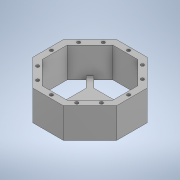
# Autodesk Inventor part: Base_Mount
Saved by Autodesk Inventor 2022 (Build 260153000, 153)
## iProperties
Created: 2022-03-21
Part Number: Base_Mount
Material: Generic
Document SubType Name: Modeling
Designer: Mlees
Density: 1 g/cm^3
Appearance: Smooth - Medium Gray
Author: Mlees
Autodesk Inventor part; units mm, degrees
ref_plane "YZ Plane" through (0, 0, 0) normal (1, 0, 0) x (0, 1, 0)
ref_plane "XZ Plane" through (0, 0, 0) normal (0, 1, 0) x (-1, 0, 0)
ref_plane "XY Plane" through (0, 0, 0) normal (0, 0, 1) x (1, 0, 0)
sketch "Sketch1" plane through (0, 0, 0) normal (0, 1, 0) x (-1, 0, 0)
  line L0 (44, -4) -> (44, -38.5)
  line L1 (38.5, -44) -> (3.5, -44)
  line L2 (-1.5, -38.5) -> (-1.5, -4)
  line L3 (4, 1.5) -> (38.5, 1.5)
  line L4 (-41.5, -44) -> (-1.5, -84)
  line L5 (-1.5, -84) -> (44, -84)
  line L6 (84, -44) -> (44, -84)
  line L7 (-41.5, 1.5) -> (-1.5, 41.5)
  line L8 (-1.5, 41.5) -> (44, 41.5)
  line L9 (84, 1.5) -> (44, 41.5)
  line L10 (-41.5, 1.5) -> (-41.5, -44)
  line L11 (84, 1.5) -> (84, -44)
  line L12 (39.8579, 31.5) -> (2.6421, 31.5)
  line L13 (-31.5, -2.6421) -> (-31.5, -39.8579)
  line L14 (2.6421, -74) -> (39.8579, -74)
  line L15 (74, -39.8579) -> (74, -2.6421)
  line L16 (38.5, 1.5) -> (54.1789, 17.1789)
  line L17 (44, -4) -> (59.6789, 11.6789)
  line L18 (44, -38.5) -> (59.6789, -54.1789)
  line L19 (38.5, -44) -> (54.1789, -59.6789)
  line L20 (3.5, -44) -> (-11.6789, -59.6789)
  line L21 (-1.5, -38.5) -> (-17.1789, -54.1789)
  line L22 (-1.5, -4) -> (-17.1789, 11.6789)
  line L23 (4, 1.5) -> (-11.6789, 17.1789)
  line L24 (74, -2.6421) -> (59.6789, 11.6789)
  line L25 (54.1789, 17.1789) -> (39.8579, 31.5)
  line L26 (39.8579, -74) -> (54.1789, -59.6789)
  line L27 (59.6789, -54.1789) -> (74, -39.8579)
  line L28 (-31.5, -39.8579) -> (-17.1789, -54.1789)
  line L29 (-11.6789, -59.6789) -> (2.6421, -74)
  line L30 (2.6421, 31.5) -> (-11.6789, 17.1789)
  line L31 (-17.1789, 11.6789) -> (-31.5, -2.6421)
  dimension "d38" = 45.5
  dimension "d39" = 45.5
  dimension "d40" = 40
  dimension "d41" = 40
  dimension "d42" = 40
  dimension "d43" = 40
  dimension "d44" = 45.5
  constraints: 64 end point, 11 perpendicular, 7 point on line, 2 parallel, 1 vertical
  measures "d38" distance of L9.start L6.start
  measures "d39" distance of L8.start L9.end
  measures "d40" distance from line of L9.start L8
  measures "d41" horizontal distance of L9.end L9.start
  measures "d42" horizontal distance of L5.end L6.start
  measures "d43" horizontal distance of L6.start L5.end
  measures "d44" distance of L4.end L5.end
extrude "Extrusion1" add sketch "Sketch1" along normal blind 5
sketch "Sketch2" plane through (0, 5, 0) normal (0, 1, 0) x (1, 0, 0)
  line L0 (-84, 44) -> (-84, -1.5) projected
  line L1 (-44, -41.5) -> (-84, -1.5)
  line L2 (-44, 84) -> (-84, 44) projected
  line L3 (-84, -1.5) -> (-84, 44)
  line L4 (-84, 44) -> (-44, 84)
  line L5 (1.5, 84) -> (-44, 84) projected
  line L6 (-44, 84) -> (1.5, 84)
  line L7 (41.5, 44) -> (1.5, 84) projected
  line L8 (1.5, 84) -> (41.5, 44)
  line L9 (41.5, -1.5) -> (41.5, 44) projected
  line L10 (41.5, 44) -> (41.5, -1.5)
  line L11 (1.5, -41.5) -> (41.5, -1.5) projected
  line L12 (41.5, -1.5) -> (1.5, -41.5)
  line L13 (-44, -41.5) -> (1.5, -41.5) projected
  line L14 (1.5, -41.5) -> (-44, -41.5)
  line L15 (-74, 2.6421) -> (-39.8579, -31.5)
  line L16 (-39.8579, -31.5) -> (-2.6421, -31.5)
  line L17 (-2.6421, -31.5) -> (31.5, 2.6421)
  line L18 (31.5, 2.6421) -> (31.5, 39.8579)
  line L19 (31.5, 39.8579) -> (-2.6421, 74)
  line L20 (-2.6421, 74) -> (-39.8579, 74)
  line L21 (-39.8579, 74) -> (-74, 39.8579)
  line L22 (-74, 39.8579) -> (-74, 2.6421)
  point P0 (0, 0)
  dimension "d22" = 10
  constraints: 32 end point, 6 collinear, 1 vertical, 7 other
  measures "d22" distance between parallel lines of L1 L15
extrude "Extrusion2" add sketch "Sketch2" along normal blind 40
sketch "Sketch4" plane through (0, 45, 0) normal (0, 1, 0) x (1, 0, 0)
  line L0 (-2.6421, -31.5) -> (-39.8579, -31.5) projected
  line L1 (11.6789, -17.1789) -> (-2.6421, -31.5) projected
  line L2 (11.6789, -17.1789) -> (17.1789, -11.6789) projected
  line L3 (41.5, -1.5) -> (41.5, 44) projected
  line L4 (31.5, 39.8579) -> (31.5, 2.6421) projected
  line L5 (-74, 2.6421) -> (-74, 39.8579) projected
  line L6 (-84, 44) -> (-84, -1.5) projected
  line L7 (1.5, -41.5) -> (41.5, -1.5) projected
  line L8 (1.5, -41.5) -> (41.5, -1.5)
  line L9 (-2.0355, -37.9645) -> (37.9645, 2.0355)
  line L10 (-84, -1.5) -> (-44, -41.5) projected
  line L11 (1.5, -41.5) -> (-44, -41.5)
  line L12 (-79, 44) -> (-79, 0.5711)
  line L13 (-79, 0.5711) -> (-41.9289, -36.5)
  line L14 (-41.9289, -36.5) -> (-0.5711, -36.5)
  line L15 (-0.5711, -36.5) -> (37.9645, 2.0355)
  line L16 (-0.5711, -36.5) -> (8.0507, -27.8782)
  point P0 (0, 0)
  point P1 (-69, -9.4289)
  point P2 (-50.5539, -27.875)
  point P3 (-21.25, -36.5)
  point P4 (26.5, -9.4289)
  point P5 (36.5, 21.25)
  point P6 (-79, 21.25)
  point P7 (-69, 51.9289)
  point P8 (-50.5539, 70.375)
  point P9 (-21.25, 79)
  point P10 (26.5, 51.9289)
  point P11 (8.0507, 70.375)
  dimension "d45" = 5
  dimension "d46" = 12.193
  constraints: 16 end point, 2 equal length, 1 coincident, 1 horizontal, 1 point on line, 3 other
  measures "d45" distance between parallel lines of L7 L9
  measures "d46" distance of L14.end L16.end
hole "Hole1" at (-69, 45, 9.4289) at (-50.5539, 45, 27.875) at (-21.25, 45, 36.5) at (26.5, 45, 9.4289) at (36.5, 45, -21.25) at (-79, 45, -21.25) at (-69, 45, -51.9289) at (-50.5539, 45, -70.375) at (-21.25, 45, -79) at (26.5, 45, -51.9289) at (8.0507, 45, 27.8782) at (8.0507, 45, -70.375) direction (0, -1, 0) diameter 4.9 depth 6 tip angle 118
body "Solid1"
